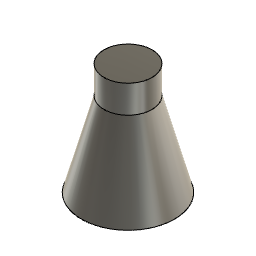
2d sketch v2 (Autodesk Fusion 360 design; units mm, degrees)
Autodesk Fusion 360 part; units mm, degrees
sketch "Sketch1" plane through (0, 0, 0) normal (0, 1, 0) x (1, 0, 0)
sketch "Sketch2" plane through (0, 0, 0) normal (0, 1, 0) x (1, 0, 0)
  line L0 (0, 0) -> (0, -180)
  line L1 (0, 0) -> (75, 0)
  line L2 (75, 0) -> (38.7653, -135.2296)
  line L3 (38.7653, -135.2296) -> (38.7653, -180)
  line L4 (0, -180) -> (38.7653, -180)
  dimension "d1" = 180
  dimension "d2" = 75
  dimension "d3" = 75
  dimension "d4" = 140
  constraint coincident L0.start L1.start
  constraint vertical L0
  constraint perpendicular L0 L1
  constraint perpendicular L1 L3
  constraint horizontal L4
  measures "d1" distance of L0.start L0.end
  measures "d2" distance of L0.start L1.end
  measures "d3" angle of L1 L2
  measures "d4" distance of L1.end L2.end
revolve "Revolve1" add sketch "Sketch2" angle 360 about axis through (0, 0, 0) along (0, 0, 1)
